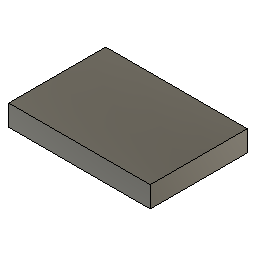
Main Body Design (Autodesk Fusion 360 archive; units mm, degrees)
design "Litium Ion Polymer Batter - 3.7V, 420 mAh"
Autodesk Fusion 360 part; units mm, degrees
sketch "Sketch1" plane through (0, 0, 0) normal (0, 0, 1) x (1, 0, 0)
  line L0 (-17.5, 12) -> (17.5, 12)
  line L1 (17.5, 12) -> (17.5, -12)
  line L2 (17.5, -12) -> (-17.5, -12)
  line L3 (-17.5, -12) -> (-17.5, 12)
  line L4 (0, 1.75) -> (0, 22.5)
  line L5 (1.75, 0) -> (22.5, 0)
  dimension "d1" = 35
  dimension "d2" = 24
  constraint horizontal L0
  constraint vertical L1
  constraint horizontal L2
  constraint vertical L3
  constraint symmetric L1 L3 L4
  constraint symmetric L0 L2 L5
  measures "d1" distance of L0.start L0.end
  measures "d2" distance of L0.end L1.end
extrude "Extrude1" add sketch "Sketch1" along normal blind 5.2
